Autodesk Inventor part; units mm, degrees
(part 2 of 2)
sketch "Эскиз15" plane through (-9.6805, -10, 23.2517) normal (0.0021195, 0, -0.9999978) x (-0.9999978, 0, -0.0021195)
  line L0 (-9.0554, 6.8747) -> (0, 6.8747) projected
  line L1 (0, 0) -> (-9.0554, 0) projected
  line L2 (0, 6.8747) -> (0, 0) projected
  line L3 (-9.0554, 6.8747) -> (0, 6.8747) projected
  line L4 (-9.0554, 0) -> (-9.0554, 6.8747) projected
  point P0 (-9.6312, 10)
  point P1 (0, 6.8747)
extrude "Выдавливание14" cut sketch "Эскиз15" against normal blind 1
sketch "Эскиз16" plane through (-0.6771, -3.1253, 47.8094) normal (0.9999978, 0, 0.0021195) x (0.0021195, 0, -0.9999978)
  line L0 (0, 0) -> (0, 14.0669) projected
  line L1 (23.5386, 0) -> (0, 0) projected
  line L2 (7.7784, 0) -> (0, 14.0669)
  point P0 (47.8108, 3.1253)
  constraints: 2 end point, 1 other
ref_plane "РабПлоскость6" through (-20.0626, 1.6111, 45.5891) normal (0.5, 0, 0.8660254) x (0.8660254, 0, -0.5)
extrude "Выдавливание15" add sketch "Эскиз16" against normal up to surface surface through (-20.0626, 1.6111, 45.5891) normal (0.5, 0, 0.8660254)
sketch "Эскиз17" plane through (-66.4, -10, 11.3065) normal (-0.9999978, 0, -0.0021195) x (-0.0021195, 0, 0.9999978)
  line L0 (36.3635, 20.9416) -> (36.3635, 6.8747) projected
  line L1 (0, 6.8747) -> (36.3635, 6.8747) projected
  line L2 (28.6929, 6.8747) -> (36.3635, 20.9416)
  point P0 (-11.4473, 10)
  constraints: 2 end point, 1 other
ref_plane "РабПлоскость7" through (-56.7244, -3.388, 39.9684) normal (-0.5, 0, 0.8660254) x (0.8660254, 0, 0.5)
extrude "Выдавливание16" add sketch "Эскиз17" along normal up to surface surface through (-56.7244, -3.388, 39.9684) normal (-0.5, 0, 0.8660254)
equation "\"Радиус_гибки\" = Толщина"
equation "\"Ширина_просечки\" = Толщина"
equation "\"Глубина_просечки\" = 0.5 * Толщина"
equation "\"Размер_просечки\" = 4 * Толщина"
equation "\"Мин_остаток\" = 2 * Толщина"
equation "\"Радиус_перехода\" = Радиус_гибки"
equation "\"Радиус_Якоби\" = Радиус_гибки"
equation "\"Размер_зазора\" = Толщина"
equation "\"Толщина\" = 3.048"
